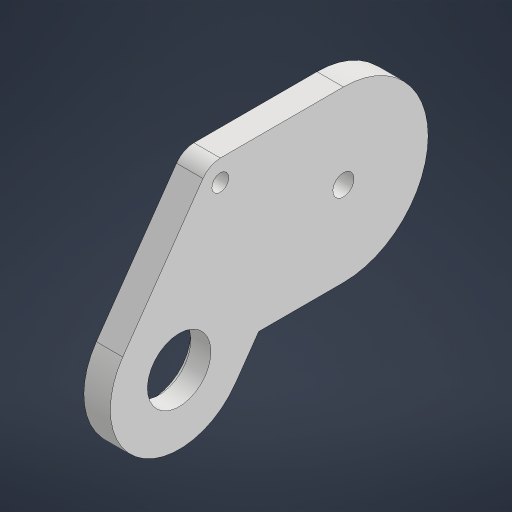
# Autodesk Inventor part: GearCover
Saved by Autodesk Inventor 2024.2 (Build 282272000, 272)
## iProperties
Created: 2023-12-29
Part Number: GearCover
Material: 一般
Document SubType Name: Modeling
Designer: Hanaoka
Density: 1 g/cm^3
Appearance: 既定
Author: Hanaoka
Autodesk Inventor part; units mm, degrees
ref_plane "YZ Plane" through (0, 0, 0) normal (1, 0, 0) x (0, 1, 0)
ref_plane "XZ Plane" through (0, 0, 0) normal (0, 1, 0) x (-1, 0, 0)
ref_plane "XY Plane" through (0, 0, 0) normal (0, 0, 1) x (1, 0, 0)
sketch "スケッチ1" plane through (0, 0, 0) normal (1, 0, 0) x (0, 1, 0)
  circle A0 centre (-7.3939, 15.5106) radius 3.6
  circle A1 centre (-7.3939, 15.5106) radius 3
  arc A2 (-3.6657, 20.8351) -> (-11.1221, 10.1862) centre (-7.3939, 15.5106) ccw
  line L0 (-11.1221, 10.1862) -> (-8, 8)
  line L1 (-8, 8) -> (-8, 0)
  line L2 (8, 0) -> (8, 11.6256)
  line L3 (7.1472, 13.2639) -> (-3.6657, 20.8351)
  circle A3 centre (-7.3939, 15.5106) radius 5
  circle A4 centre (-0.8407, 10.922) radius 3
  arc A5 (8, 11.6256) -> (7.1472, 13.2639) centre (6, 11.6256) ccw
  circle A6 centre (6, 11.6256) radius 0.8
  circle A7 centre (6, 11.6256) radius 2 construction
  circle A8 centre (-0.8407, 10.922) radius 1
  line L4 (-7.3939, 15.5106) -> (-0.8407, 10.922) construction
  arc A9 (-8, 0) -> (8, 0) centre (0, 0) ccw
  circle A10 centre (0, 0) radius 1
  line L5 (-8, 8) -> (-8, 0) construction
  line L6 (-8, 0) -> (0, 0) construction
  circle A11 centre (0, 0) radius 2 construction
  circle A12 centre (0.1153, 4.9987) radius 3
  circle A13 centre (0.1153, 4.9987) radius 1
  point P0 (8, 12.6667)
  dimension "d0" = 6
  dimension "d1" = 7.2
  dimension "d2" = 6.5
  dimension "d7" = 10
  dimension "d9" = 2
  dimension "d10" = 1.6
  dimension "d11" = 4
  dimension "d12" = 2
  dimension "d13" = 125
  dimension "d14" = 8
  dimension "d15" = 2
  dimension "d18" = 13.2
  dimension "d19" = 8
  dimension "d20" = 8
  dimension "d21" = 4
  dimension "d22" = 6
  constraints: 14 centre point, 14 end point, 10 coincident, 9 tangent, 6 point on circle, 3 parallel, 2 equal radius, 2 point on line, 1 perpendicular, 1 vertical
  measures "d0" diameter of A1
  measures "d1" diameter of A0
  measures "d2" radius of A2
  measures "d7" diameter of A3
  measures "d9" radius of A5
  measures "d10" diameter of A6
  measures "d11" diameter of A7
  measures "d12" diameter of A8
  measures "d13" angle of L1 L0
  measures "d14" radius of A9
  measures "d15" diameter of A10
  measures "d18" distance of L3.start L3.end
  measures "d19" distance of L5.end L6.end
  measures "d20" distance of L0.end L5.end
  measures "d21" diameter of A11
  measures "d22" diameter of A12
extrude "押し出し1" add sketch "スケッチ1" along normal blind 2.5 contours A0 | L3 A5 L2 A9 L1 L0 A2 | A3 | A12 | A4 | A8 | A13
extrude "押し出し2" cut sketch "スケッチ1" along normal blind 0.6 contours A0
